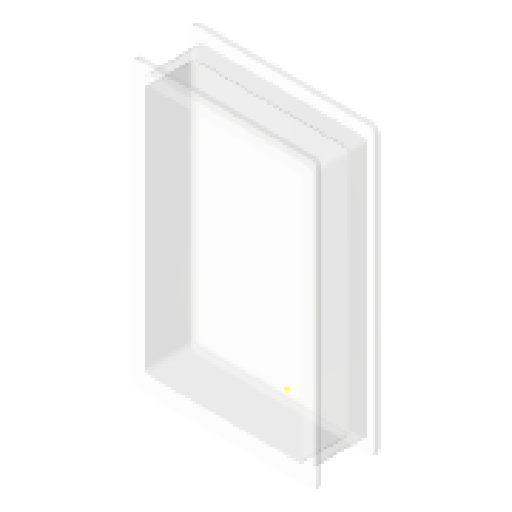
# Autodesk Inventor part: 00_Really_Useful_Box_4l_DinA4_body
Saved by Autodesk Inventor 2025.1 (Build 291241020, 241B)
## iProperties
Created: 2022-10-12
Part Number: 00_Really_Useful_Box_4l_DinA4_body
Material: Generisch
Document SubType Name: Modeling
Designer: UC2
Density: 1 g/cm^3
Appearance: Polycarbonate - Clear
Catalog Web Link: https://www.bueroshop24.de/-really-useful-box-aufbewahrungsbox-4-0-l-transparent-39-5-x-25-5-x-8-8-cm-253831?srpId=89e1a0cd4eca0f060fb9ca3bdf771869&lkz=225738&obt=0&storeType=B2C&utm_medium=psm&utm_source=idealo&utm_campaign=psm
Description: Really Useful Box Aufbewahrungsbox 4,0 l transparent 39,5 x 25,5 x 8,8 cm
Vendor: Really Useful
Mass: 2486.62 g
Surface Area: 4110.06 cm^2
Volume: 2486.62 cm^3
Author: UC2
Autodesk Inventor part; units mm, degrees
ref_plane "YZ Plane" through (0, 0, 0) normal (1, 0, 0) x (0, 1, 0)
ref_plane "XZ Plane" through (0, 0, 0) normal (0, 1, 0) x (-1, 0, 0)
ref_plane "XY Plane" through (0, 0, 0) normal (0, 0, 1) x (1, 0, 0)
sketch "Skizze1" plane through (0, 0, 0) normal (0, 0, 1) x (1, 0, 0)
  line L0 (119.5, 197.5) -> (-119.5, 197.5)
  line L1 (-127.5, 189.5) -> (-127.5, -189.5)
  line L2 (-119.5, -197.5) -> (119.5, -197.5)
  line L3 (127.5, -189.5) -> (127.5, 189.5)
  line L4 (127.5, 197.5) -> (-127.5, -197.5) construction
  line L5 (-127.5, 197.5) -> (127.5, -197.5) construction
  arc A0 (-119.5, 197.5) -> (-127.5, 189.5) centre (-119.5, 189.5) ccw
  arc A1 (127.5, 189.5) -> (119.5, 197.5) centre (119.5, 189.5) ccw
  arc A2 (119.5, -197.5) -> (127.5, -189.5) centre (119.5, -189.5) ccw
  arc A3 (-127.5, -189.5) -> (-119.5, -197.5) centre (-119.5, -189.5) ccw
  point P0 (0, 0)
  dimension "d0" = 255
  dimension "d1" = 395
  dimension "d2" = 8
  constraints: 12 end point, 8 point on circle, 8 point on line, 8 tangent, 4 centre point, 3 equal radius, 2 midpoint, 2 parallel, 1 horizontal, 1 perpendicular
  measures "d0" distance of L5.end L4.end
  measures "d1" distance of L4.end L5.start
  measures "d2" radius of A0
extrude "Extrusion1" add sketch "Skizze1" along normal blind 88
sketch "Skizze2" plane through (0, 0, 88) normal (0, 0, 1) x (1, 0, 0)
  arc A0 (-119.5, 197.5) -> (-127.5, 189.5) centre (-119.5, 189.5) ccw projected
  line L0 (-127.5, 189.5) -> (-127.5, -189.5) projected
  arc A1 (-127.5, -189.5) -> (-119.5, -197.5) centre (-119.5, -189.5) ccw projected
  line L1 (-119.5, -197.5) -> (119.5, -197.5) projected
  arc A2 (119.5, -197.5) -> (127.5, -189.5) centre (119.5, -189.5) ccw projected
  line L2 (127.5, -189.5) -> (127.5, 189.5) projected
  arc A3 (127.5, 189.5) -> (119.5, 197.5) centre (119.5, 189.5) ccw projected
  line L3 (119.5, 197.5) -> (-119.5, 197.5) projected
  line L4 (110, -174) -> (-110, -174)
  line L5 (-110, -174) -> (-110, 174)
  line L6 (-110, 174) -> (110, 174)
  line L7 (110, 174) -> (110, -174)
  line L8 (110, -174) -> (-110, 174) construction
  line L9 (-110, -174) -> (110, 174) construction
  point P0 (0, 0)
  dimension "d5" = 220
  dimension "d6" = 348
  constraints: 12 end point, 2 midpoint, 2 parallel, 1 horizontal, 1 perpendicular
  measures "d5" distance of L5.end L6.end
  measures "d6" distance of L4.end L5.end
extrude "Extrusion2" cut sketch "Skizze2" against normal blind 68 contours L4 L5 L6 L7
shell "Wandung1" thickness 7 removed faces 8 at (121.858, 197.1446, 58.6667) at (125.3644, -194.9414, 58.6667) at (39.8333, 197.5, 29.3333) at (-39.8333, -197.5, 29.3333) at (-126.4282, 193.5, 58.6667) at (-124.9414, -195.3644, 58.6667) at (-127.5, 63.1667, 58.6667) at (127.5, -63.1667, 29.3333)
sketch "Skizze3" plane through (-117, -181, 81) normal (0, -1, 0) x (1, 0, 0)
  point P0 (117, -81)
sketch "Skizze4" plane through (117, 181, 13) normal (0, 0, -1) x (-1, 0, 0)
  line L0 (234, 0) -> (0, 0) projected
  line L1 (0, 0) -> (0, -362) projected
  line L2 (0, -362) -> (234, -362) projected
  line L3 (234, -362) -> (234, 0) projected
  point P0 (117, -181)
extrude "Extrusion3" add sketch "Skizze4" along normal up to surface (13 mm away)
fillet "Rundung1" radius 8 12 edges at (117, -181, 44) (-117, -181, 44) (-110, 174, 54) (-117, 181, 44) (117, 181, 44) (110, 0, 20) (0, 174, 20) (0, -174, 20) (-110, 0, 20) (110, -174, 54) (-110, -174, 54) (110, 174, 54)
